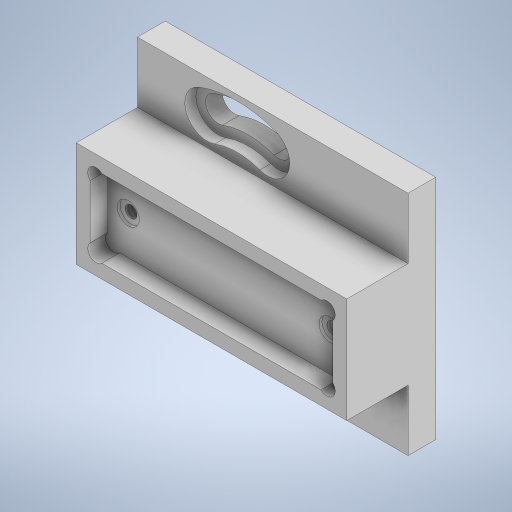
# Autodesk Inventor part: ADAPTER_AOM-brimrose
Saved by Autodesk Inventor 2024.2 (Build 282272000, 272)
## iProperties
Created: 2021-03-23
Part Number: ADAPTER_AOM-brimrose
Material: Generic
Document SubType Name: Modeling
Designer: maria
Density: 1 g/cm^3
Appearance: Default(1)
Author: maria
Autodesk Inventor part; units mm, degrees
ref_plane "YZ Plane" through (0, 0, 0) normal (1, 0, 0) x (0, 1, 0)
ref_plane "XZ Plane" through (0, 0, 0) normal (0, 1, 0) x (-1, 0, 0)
ref_plane "XY Plane" through (0, 0, 0) normal (0, 0, 1) x (1, 0, 0)
sketch "Sketch1" plane through (0, 0, 0) normal (0, 0, 1) x (1, 0, 0)
  line L0 (-24.4, -9.5) -> (24.4, -9.5)
  line L1 (24.4, -9.5) -> (24.4, 9.5)
  line L2 (24.4, 9.5) -> (-24.4, 9.5)
  line L3 (-24.4, 9.5) -> (-24.4, -9.5)
  line L4 (-24.4, -9.5) -> (24.4, 9.5) construction
  line L5 (24.4, -9.5) -> (-24.4, 9.5) construction
  point P0 (0, 0)
  dimension "LENGTH" = 48.8
  dimension "WIDTH" = 19
  constraints: 12 end point, 2 midpoint, 2 parallel, 1 horizontal, 1 perpendicular
  measures "LENGTH" distance of L1.end L2.end
  measures "WIDTH" distance of L0.end L1.end
extrude "Extrusion1" add sketch "Sketch1" along normal blind 12.85
sketch "Sketch2" plane through (0, 0, 12.85) normal (0, 0, 1) x (1, 0, 0)
  point P0 (0, 0)
  point P1 (-18.2, 0)
  point P2 (18.2, 0)
  dimension "d11" = 0
  dimension "d12" = 0
  dimension "d13" = 36.4
  dimension "d14" = 18.2
  measures "d11" vertical distance of point (-18.2, 0) point (18.2, 0)
  measures "d12" vertical distance of point (0, 0) point (-18.2, 0)
  measures "d13" distance of point (-18.2, 0) point (18.2, 0)
  measures "d14" distance of point (0, 0) point (-18.2, 0)
hole "Hole1" at (-18.2, 0, 12.85) at (18.2, 0, 12.85) direction (0, 0, -1) diameter 2.1565 depth 8.87 thread size "4-40 UNC" class "2B" standard "ANSI Unified Screw Threads"
sketch "Sketch3" plane through (0, 0, 12.85) normal (0, 0, 1) x (1, 0, 0)
  point P0 (0, 0)
  point P1 (0, 0)
  dimension "d22" = 0
  dimension "d23" = 0
  measures "d22" distance of point (0, 0) point (0, 0)
  measures "d23" distance of point (0, 0) point (0, 0)
hole "Hole2" [suppressed]
sketch "Sketch4" plane through (0, 0, 0) normal (0, 0, -1) x (-1, 0, 0)
  line L0 (5.5, 0) -> (4.5, 0) construction
  line L1 (5.5, 1.05) -> (4.5, 1.05)
  line L2 (4.5, -1.05) -> (5.5, -1.05)
  arc A0 (5.5, -1.05) -> (5.5, 1.05) centre (5.5, 0) ccw
  arc A1 (4.5, 1.05) -> (4.5, -1.05) centre (4.5, 0) ccw
  point P0 (0, 0)
  point P1 (-5, 0)
  point P2 (5, 0)
  dimension "d24" = 1
  dimension "d25" = 0
  dimension "d26" = 0
  dimension "d27" = 10
  dimension "d28" = 5
  dimension "d29" = 1.05
  constraints: 8 end point, 4 point on circle, 4 tangent, 2 centre point, 1 horizontal, 1 midpoint, 1 parallel
  measures "d24" distance of L0.start L0.end
  measures "d25" vertical distance of point (5, 0) point (-5, 0)
  measures "d26" vertical distance of point (0, 0) point (5, 0)
  measures "d27" distance of point (5, 0) point (-5, 0)
  measures "d28" distance of point (0, 0) point (5, 0)
  measures "d29" radius of A0
hole "Hole3" [suppressed]
extrude "Extrusion2" [suppressed]
sketch "Sketch5" plane through (0, 0, 0) normal (0, 0, 1) x (1, 0, 0)
  line L0 (-24.4, -20.5) -> (24.4, -20.5)
  line L1 (24.4, -20.5) -> (24.4, 20.5)
  line L2 (24.4, 20.5) -> (-24.4, 20.5)
  line L3 (-24.4, 20.5) -> (-24.4, -20.5)
  line L4 (-24.4, -20.5) -> (24.4, 20.5) construction
  line L5 (24.4, -20.5) -> (-24.4, 20.5) construction
  point P0 (0, 0)
  dimension "d39" = 48.8
  dimension "d40" = 41
  constraints: 12 end point, 2 midpoint, 2 parallel, 1 horizontal, 1 perpendicular
  measures "d39" distance of L1.end L2.end
  measures "d40" distance of L2.end L0.start
extrude "Extrusion3" add sketch "Sketch5" along normal blind 5
sketch "Sketch7" plane through (0, 0, 12.85) normal (0, 0, 1) x (1, 0, 0)
  circle A0 centre (18.2, 0) radius 1.0782 projected
  circle A1 centre (-18.2, 0) radius 1.0782 projected
  point P0 (0, 0)
  dimension "d54" = 0
  dimension "d55" = 0
  dimension "d56" = 0
  dimension "d57" = 0
  measures "d54" distance of A0.centre point (18.2, 0)
  measures "d55" distance of A0.centre point (18.2, 0)
  measures "d56" distance of A1.centre point (-18.2, 0)
  measures "d57" distance of A1.centre point (-18.2, 0)
hole "Hole5" at (18.2, 0, 12.85) at (-18.2, 0, 12.85) direction (0, 0, -1) diameter 4 depth 0.5
sketch "Sketch8" plane through (0, 0, 0) normal (0, 0, -1) x (-1, 0, 0)
  line L0 (0, 5.5) -> (0, 4.5) construction
  line L1 (-1.05, 5.5) -> (-1.05, 4.5)
  line L2 (1.05, 4.5) -> (1.05, 5.5)
  arc A0 (1.05, 5.5) -> (-1.05, 5.5) centre (0, 5.5) ccw
  arc A1 (-1.05, 4.5) -> (1.05, 4.5) centre (0, 4.5) ccw
  point P0 (0, 0)
  point P1 (0, -5)
  point P2 (0, 5)
  dimension "d77" = 1
  dimension "d78" = 1.05
  dimension "d79" = 10
  dimension "d80" = 0
  dimension "d81" = 0
  dimension "d82" = 5
  constraints: 8 end point, 4 point on circle, 4 tangent, 2 centre point, 1 midpoint, 1 parallel, 1 vertical
  measures "d77" distance of L0.start L0.end
  measures "d78" radius of A1
  measures "d79" distance of point (0, -5) point (0, 5)
  measures "d80" horizontal distance of point (0, 5) point (0, -5)
  measures "d81" horizontal distance of point (0, 0) point (0, -5)
  measures "d82" distance of point (0, 0) point (0, -5)
hole "Hole6" [suppressed]
extrude "Extrusion4" [suppressed]
sketch "Sketch10" plane through (0, 0, 12.85) normal (0, 0, 1) x (1, 0, 0)
  line L0 (-24.4, -9.5) -> (24.4, -9.5)
  line L1 (24.4, -9.5) -> (24.4, 9.5)
  line L2 (24.4, 9.5) -> (-24.4, 9.5)
  line L3 (-24.4, 9.5) -> (-24.4, -9.5)
  line L4 (-24.4, -9.5) -> (24.4, 9.5) construction
  line L5 (24.4, -9.5) -> (-24.4, 9.5) construction
  line L6 (21.9, -7) -> (-21.9, -7)
  line L7 (-21.9, -7) -> (-21.9, 7)
  line L8 (-21.9, 7) -> (21.9, 7)
  line L9 (21.9, 7) -> (21.9, -7)
  line L10 (21.9, -7) -> (-21.9, 7) construction
  line L11 (-21.9, -7) -> (21.9, 7) construction
  circle A0 centre (-20.8393, 5.9393) radius 1.5
  circle A1 centre (-20.8393, -5.9393) radius 1.5
  circle A2 centre (20.8393, 5.9393) radius 1.5
  circle A3 centre (20.8393, -5.9393) radius 1.5
  line L12 (20.8393, 5.9393) -> (21.9, 7)
  line L13 (21.9, -7) -> (20.8393, -5.9393)
  line L14 (-20.8393, 5.9393) -> (-21.9, 7)
  line L15 (-20.8393, -5.9393) -> (-21.9, -7)
  point P0 (0, 0)
  point P1 (21.9, -4.8787)
  point P2 (19.7787, -7)
  point P3 (-19.7787, -7)
  point P4 (-21.9, -4.8787)
  point P5 (-21.9, 4.8787)
  point P6 (-19.7787, 7)
  point P7 (19.7787, 7)
  point P8 (21.9, 4.8787)
  dimension "d106" = 3
  dimension "d110" = 3
  dimension "d111" = 3
  dimension "d112" = 3
  dimension "d97" = 48.8
  dimension "d98" = 19
  dimension "d99" = 43.8
  dimension "d100" = 14
  dimension "d107" = 45
  dimension "d108" = 45
  dimension "d109" = 45
  constraints: 32 end point, 4 midpoint, 4 parallel, 3 perpendicular, 2 horizontal, 12 other
  measures "d97" distance of L1.end L2.end
  measures "d98" distance of L0.end L1.end
  measures "d99" distance of L7.end L8.end
  measures "d100" distance of L8.end L6.start
  measures "d107" angle of L6 L15
  measures "d108" angle of L8 L12
  measures "d109" angle of L9 L13
extrude "Extrusion6" add sketch "Sketch10" along normal blind 3.2
chamfer "Chamfer5" [suppressed]
sketch "Sketch12" plane through (0, 0, 5) normal (0, 0, 1) x (1, 0, 0)
  arc A0 (7.9961, 15.4962) -> (-8.004, 14.5013) centre (9.4196, -136.543) ccw construction
  arc A1 (7.9587, 19.496) -> (-8.4624, 18.4749) centre (9.4196, -136.543) ccw
  arc A2 (8.0336, 11.4964) -> (-7.5457, 10.5276) centre (9.4196, -136.543) ccw
  arc A3 (8.0336, 11.4964) -> (7.9587, 19.496) centre (7.9961, 15.4962) ccw
  arc A4 (-8.4624, 18.4749) -> (-7.5457, 10.5276) centre (-8.004, 14.5013) ccw
  line L0 (24.4, 2.961) -> (24.4, -2.961)
  line L1 (24.4, 0) -> (-24.4, 0)
  line L2 (-24.4, 8.5) -> (-24.4, -8.5)
  arc A5 (7.9961, 15.4962) -> (-8.004, 14.5013) centre (9.4196, -136.543) ccw construction
  arc A6 (7.9751, 17.7461) -> (-8.2619, 16.7364) centre (9.4196, -136.543) ccw
  arc A7 (8.0172, 13.2463) -> (-7.7462, 12.2661) centre (9.4196, -136.543) ccw
  arc A8 (8.0172, 13.2463) -> (7.9751, 17.7461) centre (7.9961, 15.4962) ccw
  arc A9 (-8.2619, 16.7364) -> (-7.7462, 12.2661) centre (-8.004, 14.5013) ccw
  arc A10 (-8.004, -14.5013) -> (7.9961, -15.4962) centre (9.4196, 136.543) ccw construction
  arc A11 (-8.4624, -18.4749) -> (7.9587, -19.496) centre (9.4196, 136.543) ccw
  arc A12 (-7.5457, -10.5276) -> (8.0336, -11.4964) centre (9.4196, 136.543) ccw
  arc A13 (7.9587, -19.496) -> (8.0336, -11.4964) centre (7.9961, -15.4962) ccw
  arc A14 (-7.5457, -10.5276) -> (-8.4624, -18.4749) centre (-8.004, -14.5013) ccw
  arc A15 (-8.004, -14.5013) -> (7.9961, -15.4962) centre (9.4196, 136.543) ccw construction
  arc A16 (-8.2619, -16.7364) -> (7.9751, -17.7461) centre (9.4196, 136.543) ccw
  arc A17 (-7.7462, -12.2661) -> (8.0172, -13.2463) centre (9.4196, 136.543) ccw
  arc A18 (7.9751, -17.7461) -> (8.0172, -13.2463) centre (7.9961, -15.4962) ccw
  arc A19 (-7.7462, -12.2661) -> (-8.2619, -16.7364) centre (-8.004, -14.5013) ccw
  point P0 (0, 0)
  point P1 (-8.004, 12.753)
  point P2 (7.9961, 17.2527)
  point P3 (-6.4165, 14.3405)
  point P4 (9.5836, 18.8402)
  point P5 (-8.004, -12.753)
  point P6 (7.9961, -17.2527)
  point P7 (9.5836, -18.8402)
  point P8 (-6.4165, -14.3405)
  dimension "d118" = 8
  dimension "d122" = 4.5
  constraints: 40 point on circle, 20 centre point, 6 end point, 2 midpoint
  measures "d118" diameter of A4
  measures "d122" diameter of A9
extrude "Extrusion12" [suppressed]
extrude "Extrusion13" [suppressed]
sketch "Sketch14" plane through (0, 0, 0) normal (0, 0, -1) x (-1, 0, 0)
  point P0 (0, 0)
  point P1 (6.4, 0)
hole "Hole7" at (-6.4, 0, 0) direction (0, 0, 1) diameter 2.1 depth 2.1
sketch "Sketch15" plane through (0, 0, 0) normal (0, 0, -1) x (-1, 0, 0)
  circle A0 centre (6.4, 0) radius 1.05 projected
  circle A1 centre (6.4, 0) radius 19.5
  circle A2 centre (6.4, 0) radius 11.5
  circle A3 centre (6.4, 0) radius 17.75
  circle A4 centre (6.4, 0) radius 13.25
  line L0 (-24.4, 9.5) -> (24.4, 9.5) projected
  line L1 (24.4, 9.5) -> (-24.4, 9.5)
  line L2 (-24.4, -20.5) -> (-24.4, 20.5) projected
  line L3 (24.4, -9.5) -> (-24.4, -9.5) projected
  line L4 (24.4, -9.5) -> (-24.4, -9.5)
  arc A5 (9.3371, 17.5053) -> (5.1369, 17.705) centre (6.4, 0) ccw
  arc A6 (8.5925, 13.0673) -> (5.4572, 13.2164) centre (6.4, 0) ccw
  arc A7 (13.9857, 17.9641) -> (-1.4292, 17.8592) centre (6.4, 0) ccw
  arc A8 (10.8736, 10.5942) -> (1.7828, 10.5324) centre (6.4, 0) ccw
  arc A9 (11.8707, 14.5025) -> (0.9294, 14.5025) centre (6.4, 0) ccw construction
  arc A10 (13.2825, 18.2451) -> (-0.4824, 18.2451) centre (6.4, 0) ccw
  arc A11 (10.4589, 10.7599) -> (2.3412, 10.7599) centre (6.4, 0) ccw
  arc A12 (10.4589, 10.7599) -> (13.2825, 18.2451) centre (11.8707, 14.5025) ccw
  arc A13 (-0.4824, 18.2451) -> (2.3412, 10.7599) centre (0.9294, 14.5025) ccw
  arc A14 (11.8707, 14.5025) -> (0.9294, 14.5025) centre (6.4, 0) ccw construction
  arc A15 (12.6648, 16.6077) -> (0.1352, 16.6077) centre (6.4, 0) ccw
  arc A16 (11.0766, 12.3973) -> (1.7235, 12.3973) centre (6.4, 0) ccw
  arc A17 (11.0766, 12.3973) -> (12.6648, 16.6077) centre (11.8707, 14.5025) ccw
  arc A18 (0.1352, 16.6077) -> (1.7235, 12.3973) centre (0.9294, 14.5025) ccw
  line L5 (24.4, 9.5) -> (24.4, -9.5) projected
  line L6 (24.4, 0) -> (-24.4, 0)
  arc A19 (5.1369, -17.705) -> (9.3371, -17.5053) centre (6.4, 0) ccw
  arc A20 (5.4572, -13.2164) -> (8.5925, -13.0673) centre (6.4, 0) ccw
  arc A21 (-1.4292, -17.8592) -> (13.9857, -17.9641) centre (6.4, 0) ccw
  arc A22 (1.7828, -10.5324) -> (10.8736, -10.5942) centre (6.4, 0) ccw
  arc A23 (0.9294, -14.5025) -> (11.8707, -14.5025) centre (6.4, 0) ccw construction
  arc A24 (-0.4824, -18.2451) -> (13.2825, -18.2451) centre (6.4, 0) ccw
  arc A25 (2.3412, -10.7599) -> (10.4589, -10.7599) centre (6.4, 0) ccw
  arc A26 (13.2825, -18.2451) -> (10.4589, -10.7599) centre (11.8707, -14.5025) ccw
  arc A27 (2.3412, -10.7599) -> (-0.4824, -18.2451) centre (0.9294, -14.5025) ccw
  arc A28 (0.9294, -14.5025) -> (11.8707, -14.5025) centre (6.4, 0) ccw construction
  arc A29 (0.1352, -16.6077) -> (12.6648, -16.6077) centre (6.4, 0) ccw
  arc A30 (1.7235, -12.3973) -> (11.0766, -12.3973) centre (6.4, 0) ccw
  arc A31 (12.6648, -16.6077) -> (11.0766, -12.3973) centre (11.8707, -14.5025) ccw
  arc A32 (1.7235, -12.3973) -> (0.1352, -16.6077) centre (0.9294, -14.5025) ccw
  point P0 (0, 0)
  point P1 (-24.4, -19.5)
  point P2 (-24.4, 19.5)
  point P3 (24.4, 8.5)
  point P4 (24.4, -8.5)
  point P5 (6.4, 15.5)
  point P6 (6.4, -15.5)
  dimension "d140" = 39
  dimension "d141" = 23
  dimension "d142" = 35.5
  dimension "d143" = 26.5
  dimension "d147" = 8
  dimension "d148" = 4.5
  constraints: 58 point on circle, 32 centre point, 18 symmetric about line, 13 coincident, 8 tangent, 6 end point, 4 concentric, 2 midpoint, 1 collinear, 1 horizontal, 1 point on line, 14 other
  measures "d140" diameter of A1
  measures "d141" diameter of A2
  measures "d142" diameter of A3
  measures "d143" diameter of A4
  measures "d147" diameter of A12
  measures "d148" diameter of A17
sketch "Sketch17" plane through (0, 0, 5) normal (0, 0, 1) x (1, 0, 0)
  circle A0 centre (-6.4, 0) radius 1.05 projected
  arc A1 (-11.8725, -14.4958) -> (-0.9318, -14.4974) centre (-6.4, 0) ccw construction
  arc A2 (-12.6672, -16.6008) -> (-0.1378, -16.6026) centre (-6.4, 0) ccw
  arc A3 (-11.0779, -12.3908) -> (-1.7259, -12.3922) centre (-6.4, 0) ccw
  arc A4 (-11.0779, -12.3908) -> (-12.6672, -16.6008) centre (-11.8725, -14.4958) ccw
  arc A5 (-0.1378, -16.6026) -> (-1.7259, -12.3922) centre (-0.9318, -14.4974) ccw
  arc A6 (-11.8725, -14.4958) -> (-0.9318, -14.4974) centre (-6.4, 0) ccw construction
  arc A7 (-13.2853, -18.238) -> (0.4798, -18.24) centre (-6.4, 0) ccw
  arc A8 (-10.4598, -10.7536) -> (-2.3435, -10.7548) centre (-6.4, 0) ccw
  arc A9 (-10.4598, -10.7536) -> (-13.2853, -18.238) centre (-11.8725, -14.4958) ccw
  arc A10 (0.4798, -18.24) -> (-2.3435, -10.7548) centre (-0.9318, -14.4974) ccw
  line L0 (-24.1444, 0) -> (24.3913, 0)
  line L1 (24.3913, 0) -> (-24.1444, 0)
  arc A11 (-0.9318, 14.4974) -> (-11.8725, 14.4958) centre (-6.4, 0) ccw construction
  arc A12 (-0.1378, 16.6026) -> (-12.6672, 16.6008) centre (-6.4, 0) ccw
  arc A13 (-1.7259, 12.3922) -> (-11.0779, 12.3908) centre (-6.4, 0) ccw
  arc A14 (-12.6672, 16.6008) -> (-11.0779, 12.3908) centre (-11.8725, 14.4958) ccw
  arc A15 (-1.7259, 12.3922) -> (-0.1378, 16.6026) centre (-0.9318, 14.4974) ccw
  arc A16 (-0.9318, 14.4974) -> (-11.8725, 14.4958) centre (-6.4, 0) ccw construction
  arc A17 (0.4798, 18.24) -> (-13.2853, 18.238) centre (-6.4, 0) ccw
  arc A18 (-2.3435, 10.7548) -> (-10.4598, 10.7536) centre (-6.4, 0) ccw
  arc A19 (-13.2853, 18.238) -> (-10.4598, 10.7536) centre (-11.8725, 14.4958) ccw
  arc A20 (-2.3435, 10.7548) -> (0.4798, 18.24) centre (-0.9318, 14.4974) ccw
  point P0 (0, 0)
  point P1 (-0.9324, -14.4958)
  point P2 (-0.9324, 14.4958)
  dimension "d149" = 4.5
  dimension "d150" = 8
  constraints: 40 point on circle, 20 centre point, 11 symmetric about line, 8 tangent, 4 end point, 3 coincident, 1 collinear, 1 horizontal, 10 other
  measures "d149" diameter of A5
  measures "d150" diameter of A10
extrude "Extrusion14" cut sketch "Sketch17" against normal through all contours A4 A3 A5 A2 | A15 A13 A14 A12
extrude "Extrusion15" cut sketch "Sketch17" against normal blind 2 contours A9 A8 A10 A7 | A20 A18 A19 A17
equation "\"d2\" = BEAM_HEIGHT - APERTURE_HEIGHT"
equation "\"d14\" = 0.5 * d13"
equation "\"d39\" = LENGTH"
equation "\"d106\" = d110"
equation "\"d111\" = d110"
equation "\"d112\" = d110"
equation "\"d97\" = LENGTH"
equation "\"d98\" = WIDTH"
equation "\"BEAM_HEIGHT\" = 19.05"
equation "\"APERTURE_HEIGHT\" = 6.2"
body "Solid1"
